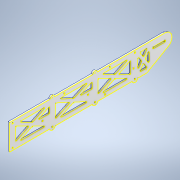
# Autodesk Inventor part: plyta_glowna_odchudzona
Saved by Autodesk Inventor 2022 (Build 260153000, 153)
## iProperties
Created: 2021-04-10
Part Number: plyta_glowna_odchudzona
Material: Aluminium 6061
Document SubType Name: Modeling
Designer: patryk.szydlik
Density: 2.7 g/cm^3
Appearance: Aluminium — płaski
Mass: 531.743 g
Surface Area: 1004.37 cm^2
Volume: 196.942 cm^3
Author: patryk.szydlik
Autodesk Inventor part; units mm, degrees
(part 1 of 2)
ref_plane "YZ Plane" through (0, 0, 0) normal (1, 0, 0) x (0, 1, 0)
ref_plane "XZ Plane" through (0, 0, 0) normal (0, 1, 0) x (-1, 0, 0)
ref_plane "XY Plane" through (0, 0, 0) normal (0, 0, 1) x (1, 0, 0)
sketch "Sketch2" plane through (0, 0, 0) normal (1, 0, 0) x (0, 1, 0)
  line L0 (127.2876, 96.9132) -> (-12.7124, 96.9132) construction
  line L1 (-12.7124, 96.9132) -> (-12.7124, -363.0868) construction
  line L2 (-12.7124, -363.0868) -> (127.2876, -363.0868) construction
  line L3 (127.2876, -363.0868) -> (127.2876, 96.9132) construction
  line L4 (97.2876, 66.9132) -> (17.2876, 66.9132) construction
  line L5 (17.2876, 66.9132) -> (17.2876, -333.0868) construction
  line L6 (17.2876, -333.0868) -> (97.2876, -333.0868) construction
  line L7 (97.2876, -333.0868) -> (97.2876, 66.9132) construction
  point P0 (0, 0)
  dimension "d2" = 140
  dimension "d3" = 460
  dimension "d4" = 80
  dimension "d5" = 400
  dimension "d6" = 30
  dimension "d7" = 30
  constraints: 16 end point, 4 parallel, 2 horizontal, 2 perpendicular
  measures "d2" distance of L2.end L1.end
  measures "d3" distance of L1.end L0.end
  measures "d4" distance of L6.end L5.end
  measures "d5" distance of L5.end L4.end
  measures "d6" distance between parallel lines of L3 L7
  measures "d7" distance between parallel lines of L0 L4
sketch "Sketch3" plane through (0, 0, 0) normal (1, 0, 0) x (0, 1, 0)
  circle A0 centre (-62.7124, 46.9132) radius 20
  line L0 (-12.7124, 96.9132) -> (-12.7124, -363.0868) construction
  circle A1 centre (-62.7124, -33.0868) radius 20
  circle A2 centre (-62.7124, -113.0868) radius 20
  circle A3 centre (-62.7124, -193.0868) radius 20
  circle A4 centre (-62.7124, -273.0868) radius 20
  circle A5 centre (-62.7124, -353.0868) radius 20
  line L1 (127.2876, 96.9132) -> (-12.7124, 96.9132) construction
  point P0 (0, 0)
  dimension "d8" = 40
  dimension "d9" = 50
  dimension "d12" = 80
  dimension "d17" = 50
  constraints: 6 centre point, 1 vertical, 10 other
  measures "d8" diameter of A0
  measures "d9" distance from line of L0 A0.centre
  measures "d12" distance of A0.centre A1.centre
  measures "d17" distance from line of A0.centre L1
sketch "Sketch1" plane through (0, 0, 0) normal (1, 0, 0) x (0, 1, 0)
  circle A0 centre (65.5719, 146.9132) radius 40
  circle A1 centre (65.5719, -453.0868) radius 40
  line L0 (127.2876, 96.9132) -> (-12.7124, 96.9132) construction
  line L1 (-12.7124, -363.0868) -> (127.2876, -363.0868) construction
  line L2 (-62.7124, 46.9132) -> (-62.7124, -33.0868) construction
  line L3 (-62.7124, -273.0868) -> (-62.7124, -353.0868) construction
  line L4 (105.2399, 141.7706) -> (105.5719, -453.0645) construction
  circle A2 centre (-62.7124, 46.9132) radius 20 projected
  line L5 (37.2876, 175.1975) -> (-76.8545, 61.0553)
  circle A3 centre (-62.7124, -353.0868) radius 20 projected
  line L6 (-76.8545, -367.2289) -> (37.2876, -481.3711) construction
  point P0 (0, 0)
  dimension "d0" = 80
  dimension "d1" = 80
  dimension "d18" = 50
  dimension "d19" = 90
  dimension "d45" = 135
  dimension "d46" = 135
  constraints: 10 end point, 4 point on circle, 3 tangent, 2 centre point, 2 coincident, 2 vertical, 6 other
  measures "d0" diameter of A0
  measures "d1" diameter of A1
  measures "d18" distance from line of A0.centre L0
  measures "d19" distance from line of A1.centre L1
  measures "d45" angle of L2 L5
  measures "d46" angle of L3 L6
sketch "Sketch4" plane through (0, 0, 0) normal (1, 0, 0) x (0, 1, 0)
  line L0 (37.6815, -23.0868) -> (-57.7124, 6.9132) construction
  circle A0 centre (-62.7124, 46.9132) radius 20 projected
  circle A1 centre (-62.7124, -33.0868) radius 20 projected
  line L1 (-62.7124, 46.9132) -> (-62.7124, -33.0868) construction
  circle A2 centre (-27.7124, 92.5679) radius 20 construction
  circle A3 centre (-27.7124, 12.5679) radius 20 construction
  line L2 (-27.7124, 52.5679) -> (37.6815, -23.0868) construction
  line L3 (-27.7124, 52.5679) -> (-57.7124, 6.9132) construction
  line L4 (37.6815, -23.0868) -> (-42.7124, 29.7406) construction
  line L5 (-12.7124, 96.9132) -> (-12.7124, -363.0868) construction
  point P0 (0, 0)
  point P1 (-61.7124, 47.9132)
  point P2 (83.0715, 59.9132)
  point P3 (83.0715, -100.0868)
  point P4 (37.6815, -183.0868)
  point P5 (83.0715, -260.0868)
  point P6 (37.6815, -343.0868)
  dimension "d22" = 40
  dimension "d23" = 5
  dimension "d24" = 30
  dimension "d25" = 40
  dimension "d26" = 40
  dimension "d27" = 80
  dimension "d28" = 40
  dimension "d29" = 100
  dimension "d30" = 100
  dimension "d31" = 35
  dimension "d32" = 54.6292
  dimension "d33" = 27.3146
  dimension "d34" = 56.691
  dimension "d35" = 95.3939
  dimension "d36" = 45.39
  dimension "d37" = 83
  dimension "d40" = 160
  constraints: 8 end point, 2 centre point, 2 vertical alignment, 1 coincident, 1 midpoint, 1 vertical, 4 other
  measures "d22" vertical distance of point (-62.712, 46.913) L0.end
  measures "d23" horizontal distance of point (-62.712, 46.913) L0.end
  measures "d24" vertical distance of L0.end L0.start
  measures "d25" diameter of A3
  measures "d26" diameter of A2
  measures "d27" distance of A3.centre A2.centre
  measures "d28" distance of A3.centre L2.start
  measures "d29" distance of L0.start L0.end
  measures "d30" distance of L2.start L0.start
  measures "d31" horizontal distance of point (-62.712, 46.913) A2.centre
  measures "d32" distance of L0.end L2.start
  measures "d33" distance of L0.end L4.end
  measures "d34" angle of L5 L4
  measures "d35" horizontal distance of L0.end L0.start
  measures "d36" horizontal distance of L0.start point (83.072, 59.913)
  measures "d37" vertical distance of L0.start point (83.072, 59.913)
  measures "d40" distance of point (83.072, 59.913) point (83.072, -100.087)
sketch "Sketch6" plane through (0, 0, 0) normal (1, 0, 0) x (0, 1, 0)
  line L0 (234.6261, -208.0868) -> (-157.479, -208.0868) construction
  line L1 (237.7494, -58.0868) -> (-154.3557, -58.0868) construction
  line L2 (17.2876, -333.0868) -> (97.2876, -333.0868) construction
  line L3 (97.2876, 66.9132) -> (17.2876, 66.9132) construction
  point P0 (0, 0)
  dimension "d61" = 125
  dimension "d62" = 125
  constraints: 4 end point, 2 horizontal
  measures "d61" distance between parallel lines of L1 L3
  measures "d62" distance between parallel lines of L2 L0
sketch "Sketch5" plane through (0, 0, 0) normal (1, 0, 0) x (0, 1, 0)
  arc A0 (90.5719, 146.9132) -> (47.8942, 164.5909) centre (65.5719, 146.9132) ccw
  arc A1 (90.5719, -453.0868) -> (43.9213, -465.5868) centre (65.5719, -453.0868) ccw construction
  line L0 (90.5719, -453.0868) -> (90.5719, 146.9132)
  arc A2 (30.1815, -170.0964) -> (23.5862, -188.2171) centre (37.6815, -183.0868) ccw
  arc A3 (30.1815, -330.0964) -> (23.5862, -348.2171) centre (37.6815, -343.0868) ccw
  arc A4 (30.1815, -10.0964) -> (22.6815, -23.0868) centre (37.6815, -23.0868) ccw
  line L1 (30.1815, -170.0964) -> (40.5719, -164.0975) construction
  line L2 (30.1815, -10.0964) -> (40.5719, -4.0975) construction
  circle A5 centre (83.0715, -100.0868) radius 12.5 construction
  circle A6 centre (83.0715, -260.0868) radius 12.5 construction
  circle A7 centre (83.0715, 59.9132) radius 12.5 construction
  line L3 (71.9467, 54.2134) -> (71.9467, 54.182) construction
  line L4 (72.2462, 53.6632) -> (71.9467, 54.182) construction
  line L5 (37.6815, -23.0868) -> (69.2216, -23.0868) construction
  arc A8 (47.8942, 164.5909) -> (90.5719, 146.9132) centre (65.5719, 146.9132) ccw construction
  arc A9 (40.5719, -8.3679) -> (30.1815, -10.0964) centre (37.6815, -23.0868) ccw construction
  arc A10 (40.5719, -37.8057) -> (40.5719, -8.3679) centre (37.6815, -23.0868) ccw construction
  arc A11 (22.6815, -23.0868) -> (40.5719, -37.8057) centre (37.6815, -23.0868) ccw construction
  arc A12 (40.5719, -168.3679) -> (30.1815, -170.0964) centre (37.6815, -183.0868) ccw construction
  arc A13 (40.5719, -197.8057) -> (40.5719, -168.3679) centre (37.6815, -183.0868) ccw construction
  arc A14 (23.5862, -188.2171) -> (40.5719, -197.8057) centre (37.6815, -183.0868) ccw construction
  arc A15 (40.5719, -328.3679) -> (30.1815, -330.0964) centre (37.6815, -343.0868) ccw construction
  arc A16 (23.5862, -348.2171) -> (40.5719, -328.3679) centre (37.6815, -343.0868) ccw construction
  arc A17 (43.9213, -465.5868) -> (90.5719, -453.0868) centre (65.5719, -453.0868) ccw
  arc A18 (62.5719, -453.0868) -> (68.5719, -453.0868) centre (65.5719, -453.0868) ccw
  arc A19 (68.5719, -413.0868) -> (62.5719, -413.0868) centre (65.5719, -413.0868) ccw
  line L6 (68.5719, -413.0868) -> (68.5719, -453.0868)
  line L7 (62.5719, -413.0868) -> (62.5719, -453.0868)
  arc A20 (68.5719, -453.0868) -> (62.5719, -453.0868) centre (65.5719, -453.0868) ccw construction
  arc A21 (62.5719, -413.0868) -> (68.5719, -413.0868) centre (65.5719, -413.0868) ccw construction
  line L8 (127.2876, 96.9132) -> (-12.7124, 96.9132) construction
  line L9 (-12.7124, -363.0868) -> (127.2876, -363.0868) construction
  line L10 (237.7494, -58.0868) -> (-154.3557, -58.0868) construction
  line L11 (234.6261, -208.0868) -> (-157.479, -208.0868) construction
  circle A22 centre (65.5719, 146.9132) radius 11
  circle A23 centre (65.5719, -413.0868) radius 50 construction
  circle A24 centre (65.5719, 146.9132) radius 55 construction
  line L12 (0.5719, 117.2685) -> (47.8942, 164.5909)
  line L13 (43.9213, -465.5868) -> (0.5719, -390.5035)
  line L14 (0.5719, -390.5035) -> (0.5719, 117.2685)
  line L15 (17.2876, 66.9132) -> (17.2876, -333.0868) construction
  circle A25 centre (2.2876, -58.0868) radius 10
  circle A26 centre (2.2876, -348.0868) radius 10
  circle A27 centre (2.2876, -208.0868) radius 10
  circle A28 centre (90.5719, -208.0868) radius 7.5
  circle A29 centre (90.5719, -58.0868) radius 7.5
  point P0 (0, 0)
  point P1 (71.9467, -17.6422)
  point P2 (71.9467, -177.6422)
  point P3 (71.9467, -268.3281)
  point P4 (71.9467, -337.6422)
  point P5 (83.0719, 81.9132)
  point P6 (83.0719, -348.0868)
  point P7 (83.0719, -366.2493)
  point P8 (16.3278, 122.4179)
  point P9 (16.56, -403.1957)
  point P10 (8.0719, -82.4742)
  point P11 (8.0719, -243.0868)
  point P12 (0.5719, -338.2351)
  point P13 (0.5719, -357.9385)
  point P14 (0.5719, -48.2351)
  point P15 (0.5719, -67.9385)
  point P16 (0.5719, -198.2351)
  point P17 (0.5719, -217.9385)
  point P18 (8.0719, 81.9132)
  point P19 (90.5719, -200.5868)
  point P20 (90.5719, -215.5868)
  point P21 (90.5719, -50.5868)
  point P22 (90.5719, -65.5868)
  dimension "d84" = 110
  dimension "d47" = 50
  dimension "d48" = 50
  dimension "d49" = 30
  dimension "d50" = 30
  dimension "d51" = 30
  dimension "d52" = 25
  dimension "d54" = 25
  dimension "d58" = 6
  dimension "d59" = 6
  dimension "d60" = 40
  dimension "d63" = 15
  dimension "d64" = 7.5
  dimension "d65" = 15
  dimension "d66" = 7.5
  dimension "d81" = 22
  dimension "d82" = 100
  dimension "d86" = 90
  dimension "d92" = 7.5
  dimension "d101" = 7.5
  dimension "d102" = 7.5
  dimension "d103" = 135
  dimension "d104" = 150
  dimension "d139" = 7.5004
  dimension "d141" = 0
  dimension "d142" = 0
  dimension "d145" = 25
  dimension "d150" = 15
  dimension "d151" = 15
  dimension "d152" = 20
  dimension "d153" = 20
  dimension "d154" = 20
  dimension "d155" = 15
  dimension "d159" = 15
  dimension "d160" = 7.5
  dimension "d161" = 15
  dimension "d162" = 15
  constraints: 45 point on circle, 29 centre point, 22 end point, 18 coincident, 8 point on line, 8 tangent, 4 vertical, 2 vertical alignment, 1 horizontal, 1 horizontal alignment, 3 other
  measures "d47" diameter of A0
  measures "d48" diameter of A1
  measures "d49" diameter of A2
  measures "d50" diameter of A3
  measures "d51" diameter of A4
  measures "d52" diameter of A5
  measures "d54" diameter of A7
  measures "d58" diameter of A18
  measures "d59" diameter of A19
  measures "d60" distance of point (65.572, -453.087) point (65.572, -413.087)
  measures "d63" distance from line of L8 point (83.072, 81.913)
  measures "d64" distance from line of L0 point (83.072, 81.913)
  measures "d65" distance from line of L9 point (83.072, -348.087)
  measures "d66" distance from line of L0 point (83.072, -348.087)
  measures "d81" diameter of A22
  measures "d82" diameter of A23
  measures "d86" distance between parallel lines of L14 L0
  measures "d92" distance from line of L0 A23.start
  measures "d101" distance from line of point (16.328, 122.418) L12
  measures "d102" distance from line of L13 A23.end
  measures "d103" angle of L12 L14
  measures "d104" angle of L14 L13
  measures "d139" distance from line of L0 point (83.072, -100.087)
  measures "d141" distance from line of L0 point (90.572, -58.087)
  measures "d142" distance from line of L0 point (90.572, -208.087)
  measures "d145" diameter of A6
  measures "d150" distance from line of point (2.288, -348.087) L15
  measures "d151" distance from line of L15 point (2.288, -58.087)
  measures "d152" diameter of A25
  measures "d153" diameter of A26
  measures "d154" diameter of A27
  measures "d155" distance from line of L15 point (2.288, -208.087)
  measures "d159" distance from line of L8 point (8.072, 81.913)
  measures "d160" distance from line of L14 point (8.072, 81.913)
  measures "d161" diameter of A28
  measures "d162" diameter of A29
extrude "Extrusion1" add sketch "Sketch5" against normal blind 5
hole "Hole1" at (0, 83.0719, 81.9132) at (0, 83.0715, 59.9132) at (0, 16.3278, 122.4179) at (0, 37.6815, -23.0868) at (0, 90.5719, -58.0868) at (0, 8.0719, -82.4742) at (0, 83.0715, -100.0868) at (0, 37.6815, -183.0868) at (0, 90.5719, -208.0868) at (0, 8.0719, -243.0868) at (0, 83.0715, -260.0868) at (0, 2.2876, -348.0868) at (0, 37.6815, -343.0868) at (0, 16.56, -403.1957) at (0, 83.0719, -348.0868) at (0, 83.0719, -366.2493) at (0, 2.2876, -58.0868) at (0, 2.2876, -208.0868) at (0, 8.0719, 81.9132) direction (-1, 0, 0) diameter 5 end through all clearance for "Flat Head Machine Screw" size "M5" standard "Ansi Metric M Profile"
sketch "Sketch7" plane through (0, 0, 0) normal (1, 0, 0) x (0, 0, -1)
  circle A0 centre (348.0868, 83.0719) radius 2.5 projected
  circle A1 centre (343.0868, 37.6815) radius 2.5 projected
  circle A2 centre (243.0868, 8.0719) radius 2.5 projected
  circle A3 centre (82.4742, 8.0719) radius 2.5 projected
  circle A4 centre (58.0868, 90.5719) radius 2.5 projected
  circle A5 centre (-122.4179, 16.3278) radius 2.5 projected
  circle A6 centre (-81.9132, 83.0719) radius 2.5 projected
  circle A7 centre (-59.9132, 83.0715) radius 2.5 projected
  circle A8 centre (23.0868, 37.6815) radius 2.5 projected
  circle A9 centre (100.0868, 83.0715) radius 2.5 projected
  circle A10 centre (183.0868, 37.6815) radius 2.5 projected
  circle A11 centre (208.0868, 90.5719) radius 2.5 projected
  circle A12 centre (260.0868, 83.0715) radius 2.5 projected
  circle A13 centre (348.0868, 2.2876) radius 2.5 projected
  circle A14 centre (403.1957, 16.56) radius 2.5 projected
  circle A15 centre (366.2493, 83.0719) radius 2.5 projected
  line L0 (-117.2685, 0.5719) -> (48.2351, 0.5719) projected
  line L1 (390.5035, 0.5719) -> (465.5868, 43.9213) projected
  arc A16 (465.5868, 43.9213) -> (453.0868, 90.5719) centre (453.0868, 65.5719) ccw projected
  line L2 (453.0868, 90.5719) -> (215.5868, 90.5719) projected
  arc A17 (-146.9132, 90.5719) -> (-164.5909, 47.8942) centre (-146.9132, 65.5719) ccw projected
  line L3 (-164.5909, 47.8942) -> (-117.2685, 0.5719) projected
  circle A18 centre (-146.9132, 65.5719) radius 11 projected
  arc A19 (453.0868, 62.5719) -> (453.0868, 68.5719) centre (453.0868, 65.5719) ccw projected
  line L4 (453.0868, 62.5719) -> (413.0868, 62.5719) projected
  arc A20 (413.0868, 68.5719) -> (413.0868, 62.5719) centre (413.0868, 65.5719) ccw projected
  line L5 (413.0868, 68.5719) -> (453.0868, 68.5719) projected
  line L6 (-146.9132, 75.5719) -> (453.0868, 75.5719)
  arc A21 (458.0868, 56.9116) -> (453.0868, 75.5719) centre (453.0868, 65.5719) ccw
  line L7 (458.0868, 56.9116) -> (386.4843, 15.5719)
  line L8 (386.4843, 15.5719) -> (398.0868, 15.5719)
  line L9 (-111.0553, 15.5719) -> (-153.9843, 58.5008)
  arc A22 (-146.9132, 75.5719) -> (-153.9843, 58.5008) centre (-146.9132, 65.5719) ccw
  line L10 (453.0868, 90.5719) -> (-146.9132, 90.5719) projected
  line L11 (-91.9132, 90.5719) -> (-71.9132, 90.5719)
  line L12 (-71.9132, 90.5719) -> (-71.9132, 0.5719)
  line L13 (-71.9132, 0.5719) -> (-91.9132, 0.5719)
  line L14 (-91.9132, 0.5719) -> (-91.9132, 90.5719)
  line L15 (-117.2685, 0.5719) -> (390.5035, 0.5719) projected
  line L16 (48.0868, 90.5719) -> (68.0868, 90.5719)
  line L17 (68.0868, 90.5719) -> (68.0868, 0.5719)
  line L18 (68.0868, 0.5719) -> (48.0868, 0.5719)
  line L19 (48.0868, 0.5719) -> (48.0868, 90.5719)
  line L20 (198.0868, 90.5719) -> (218.0868, 90.5719)
  line L21 (218.0868, 90.5719) -> (218.0868, 0.5719)
  line L22 (218.0868, 0.5719) -> (198.0868, 0.5719)
  line L23 (198.0868, 0.5719) -> (198.0868, 90.5719)
  line L24 (338.0868, 90.5719) -> (358.0868, 90.5719)
  line L25 (358.0868, 90.5719) -> (358.0868, 38.7436)
  line L26 (358.0868, 0.5719) -> (338.0868, 0.5719)
  line L27 (338.0868, 0.5719) -> (338.0868, 90.5719)
  circle A23 centre (-146.9132, 65.5719) radius 25 construction
  arc A24 (453.0868, 62.5719) -> (453.0868, 68.5719) centre (453.0868, 65.5719) ccw construction
  circle A25 centre (453.0868, 65.5719) radius 25 construction
  arc A26 (413.0868, 68.5719) -> (413.0868, 62.5719) centre (413.0868, 65.5719) ccw construction
  line L28 (-146.9132, 90.5719) -> (453.0868, 90.5719) construction
  line L29 (398.0911, 65.9314) -> (398.0911, 90.5719) construction
  line L30 (403.0868, 38.7436) -> (456.6188, 38.7436) construction
  line L31 (465.5868, 43.9213) -> (390.5035, 0.5719) construction
  line L32 (403.0868, 38.7436) -> (403.0868, 15.5719) construction
  line L33 (398.0868, 65.5719) -> (398.0868, 38.7436) construction
  line L34 (398.0868, 38.7436) -> (398.0868, 38.7436) construction
  line L35 (398.0868, 15.5719) -> (398.0868, 38.7436) construction
  line L36 (408.0868, 38.7436) -> (408.0868, 15.5719) construction
  line L37 (358.0868, 38.7436) -> (358.0868, 0.5719)
  line L38 (398.0868, 38.7436) -> (403.0868, 38.7436) construction
  line L39 (398.0868, 15.5719) -> (-111.0553, 15.5719)
  line L40 (218.0868, 75.5719) -> (338.0868, 15.5719) construction
  line L41 (218.0868, 15.5719) -> (338.0868, 75.5719) construction
  line L42 (326.9065, 75.5719) -> (218.0868, 21.1621) construction
  line L43 (229.2671, 15.5719) -> (338.0868, 69.9817) construction
  line L44 (229.2671, 75.5719) -> (338.0868, 21.1621) construction
  line L45 (218.0868, 69.9817) -> (326.9065, 15.5719) construction
  line L46 (333.0868, 67.4817) -> (333.0868, 23.6621) construction
  line L47 (68.0868, 75.5719) -> (198.0868, 15.5719) construction
  line L48 (198.0868, 75.5719) -> (68.0868, 15.5719) construction
  line L49 (68.0868, 21.0788) -> (186.1553, 75.5719) construction
  line L50 (80.0183, 15.5719) -> (198.0868, 70.065) construction
  line L51 (198.0868, 21.0788) -> (80.0183, 75.5719) construction
  line L52 (68.0868, 70.065) -> (186.1553, 15.5719) construction
  line L53 (48.0868, 15.5719) -> (-71.9132, 75.5719) construction
  line L54 (-71.9132, 15.5719) -> (48.0868, 75.5719) construction
  line L55 (36.9065, 75.5719) -> (-71.9132, 21.1621) construction
  line L56 (-60.7329, 15.5719) -> (48.0868, 69.9817) construction
  line L57 (-60.7329, 75.5719) -> (48.0868, 21.1621) construction
  line L58 (-71.9132, 69.9817) -> (36.9065, 15.5719) construction
  line L59 (68.0868, 73.0715) -> (61.5727, 73.0715) construction
  line L60 (48.0868, 47.6815) -> (-4.9522, 47.6815) construction
  line L61 (198.0868, 47.6815) -> (140.4474, 47.6815) construction
  line L62 (218.0868, 73.0715) -> (211.9072, 73.0715) construction
  line L63 (-121.9132, 65.5719) -> (-121.9132, 75.5719) construction
  line L64 (-121.9132, 65.5719) -> (-121.9132, 26.4298) construction
  line L65 (-121.9132, 75.5719) -> (-91.9132, 15.5719) construction
  line L66 (-91.9132, 26.7522) -> (-116.323, 75.5719) construction
  line L67 (-121.9132, 64.3916) -> (-97.5034, 15.5719) construction
  line L68 (-111.0553, 15.5719) -> (-121.9132, 15.5719) construction
  line L69 (-121.9132, 15.5719) -> (-121.9132, 26.4298) construction
  line L70 (-121.9132, 15.5719) -> (-91.9132, 75.5719) construction
  line L71 (-97.5034, 75.5719) -> (-121.9132, 26.7522) construction
  line L72 (-116.323, 15.5719) -> (-91.9132, 64.3916) construction
  circle A27 centre (413.0868, 65.5719) radius 15 construction
  line L73 (398.0911, 75.5719) -> (358.0868, 15.5719) construction
  line L74 (398.0868, 15.5719) -> (358.0868, 75.5719) construction
  line L75 (392.0816, 75.5719) -> (358.0868, 24.5851) construction
  line L76 (398.0911, 66.5587) -> (364.0962, 15.5719) construction
  line L77 (358.0868, 66.558) -> (392.0775, 15.5719) construction
  line L78 (398.0868, 24.5858) -> (364.096, 75.5719) construction
  circle A28 centre (58.0868, 2.2876) radius 2.5 projected
  line L79 (67.9385, 0.5719) -> (198.2351, 0.5719) projected
  line L80 (217.9385, 0.5719) -> (338.2351, 0.5719) projected
  arc A29 (48.2351, 0.5719) -> (67.9385, 0.5719) centre (58.0868, 2.2876) ccw projected
  arc A30 (338.2351, 0.5719) -> (357.9385, 0.5719) centre (348.0868, 2.2876) ccw projected
  arc A31 (198.2351, 0.5719) -> (217.9385, 0.5719) centre (208.0868, 2.2876) ccw projected
  line L81 (357.9385, 0.5719) -> (390.5035, 0.5719) projected
  line L82 (200.5868, 90.5719) -> (65.5868, 90.5719) projected
  line L83 (50.5868, 90.5719) -> (-146.9132, 90.5719) projected
  arc A32 (215.5868, 90.5719) -> (200.5868, 90.5719) centre (208.0868, 90.5719) ccw projected
  arc A33 (65.5868, 90.5719) -> (50.5868, 90.5719) centre (58.0868, 90.5719) ccw projected
  point P0 (0, 0)
  dimension "d93" = 15
  dimension "d94" = 10
  dimension "d95" = 20
  dimension "d97" = 20
  dimension "d99" = 20
  dimension "d100" = 10
  dimension "d105" = 20
  dimension "d107" = 5
  dimension "d108" = 5
  dimension "d111" = 5
  dimension "d112" = 5
  dimension "d113" = 5
  dimension "d114" = 5
  dimension "d115" = 10
  dimension "d116" = 5
  dimension "d117" = 5
  dimension "d118" = 5
  dimension "d119" = 5
  dimension "d120" = 5
  dimension "d121" = 5
  dimension "d122" = 5
  dimension "d123" = 5
  dimension "d124" = 10
  dimension "d125" = 10
  dimension "d126" = 10
  dimension "d127" = 10
  dimension "d128" = 5
  dimension "d129" = 5
  dimension "d130" = 5
  dimension "d131" = 5
  dimension "d132" = 30
  dimension "d133" = 5
  dimension "d134" = 5
  dimension "d135" = 5
  dimension "d136" = 5
  dimension "d148" = 10
  dimension "d149" = 10
  constraints: 134 end point, 61 point on line, 29 parallel, 11 perpendicular, 9 horizontal, 6 point on circle, 6 vertical, 4 centre point, 4 coincident, 1 collinear, 1 concentric, 1 horizontal alignment, 50 other
  measures "d94" distance from line of L12 A6.centre
  measures "d95" distance of L17.end L18.end
  measures "d97" distance of L21.end L22.end
  measures "d99" distance of L26.start L26.end
  measures "d100" distance from line of L25 A0.centre
  measures "d105" distance between parallel lines of L12 L14
  measures "d107" distance between parallel lines of L35 L32
  measures "d108" distance between parallel lines of L32 L36
  measures "d111" distance between parallel lines of L42 L41
  measures "d112" distance between parallel lines of L41 L43
  measures "d113" distance between parallel lines of L40 L44
  measures "d114" distance between parallel lines of L45 L40
  measures "d115" distance from line of L46 A1.centre
  measures "d116" distance between parallel lines of L50 L48
  measures "d117" distance between parallel lines of L49 L48
  measures "d118" distance between parallel lines of L51 L47
  measures "d119" distance between parallel lines of L52 L47
  measures "d120" distance between parallel lines of L57 L53
  measures "d121" distance between parallel lines of L58 L53
  measures "d122" distance between parallel lines of L54 L55
  measures "d123" distance between parallel lines of L56 L54
  measures "d124" distance from line of L59 A9.centre
  measures "d125" distance from line of L60 A8.centre
  measures "d126" distance from line of L61 A10.centre
  measures "d127" distance from line of L62 A12.centre
  measures "d128" distance between parallel lines of L65 L66
  measures "d129" distance between parallel lines of L65 L67
  measures "d130" distance between parallel lines of L72 L70
  measures "d131" distance between parallel lines of L71 L70
  measures "d132" diameter of A27
  measures "d133" distance between parallel lines of L73 L75
  measures "d134" distance between parallel lines of L76 L73
  measures "d135" distance between parallel lines of L78 L74
  measures "d136" distance between parallel lines of L77 L74
  measures "d148" distance from line of L17 A4.centre
  measures "d149" distance from line of L23 A11.centre
sketch "Sketch8" plane through (0, 0, 0) normal (1, 0, 0) x (0, 0, -1)
  line L0 (-116.323, 15.5719) -> (-91.9132, 64.3916) projected
  line L1 (-91.9132, 26.7522) -> (-116.323, 75.5719) projected
  line L2 (-91.9132, 0.5719) -> (-91.9132, 90.5719) projected
  line L3 (-121.9132, 64.3916) -> (-97.5034, 15.5719) projected
  line L4 (398.0868, 15.5719) -> (-111.0553, 15.5719) projected
  line L5 (-111.0553, 15.5719) -> (-121.9132, 15.5719) projected
  line L6 (-97.5034, 75.5719) -> (-121.9132, 26.7522) projected
  line L7 (-121.9132, 65.5719) -> (-121.9132, 26.4298) projected
  line L8 (-146.9132, 75.5719) -> (453.0868, 75.5719) projected
  line L9 (-71.9132, 69.9817) -> (36.9065, 15.5719) projected
  line L10 (-71.9132, 90.5719) -> (-71.9132, 0.5719) projected
  line L11 (36.9065, 75.5719) -> (-71.9132, 21.1621) projected
  line L12 (-60.7329, 75.5719) -> (48.0868, 21.1621) projected
  line L13 (-60.7329, 15.5719) -> (48.0868, 69.9817) projected
  line L14 (48.0868, 47.6815) -> (-4.9522, 47.6815) projected
  line L15 (48.0868, 0.5719) -> (48.0868, 90.5719) projected
  line L16 (68.0868, 73.0715) -> (61.5727, 73.0715) projected
  line L17 (68.0868, 90.5719) -> (68.0868, 0.5719) projected
  line L18 (68.0868, 21.0788) -> (186.1553, 75.5719) projected
  line L19 (80.0183, 15.5719) -> (198.0868, 70.065) projected
  line L20 (68.0868, 70.065) -> (186.1553, 15.5719) projected
  line L21 (198.0868, 21.0788) -> (80.0183, 75.5719) projected
  line L22 (198.0868, 47.6815) -> (140.4474, 47.6815) projected
  line L23 (198.0868, 0.5719) -> (198.0868, 90.5719) projected
  line L24 (218.0868, 73.0715) -> (211.9072, 73.0715) projected
  line L25 (218.0868, 69.9817) -> (326.9065, 15.5719) projected
  line L26 (326.9065, 75.5719) -> (218.0868, 21.1621) projected
  line L27 (218.0868, 90.5719) -> (218.0868, 0.5719) projected
  line L28 (229.2671, 15.5719) -> (338.0868, 69.9817) projected
  line L29 (229.2671, 75.5719) -> (338.0868, 21.1621) projected
  line L30 (333.0868, 67.4817) -> (333.0868, 23.6621) projected
  line L31 (358.0868, 66.558) -> (392.0775, 15.5719) projected
  line L32 (392.0816, 75.5719) -> (358.0868, 24.5851) projected
  line L33 (358.0868, 90.5719) -> (358.0868, 38.7436) projected
  line L34 (358.0868, 38.7436) -> (358.0868, 0.5719) projected
  line L35 (398.0911, 66.5587) -> (364.0962, 15.5719) projected
  line L36 (398.0868, 24.5858) -> (364.096, 75.5719) projected
  line L37 (398.0868, 65.5719) -> (398.0868, 38.7436) projected
  line L38 (398.0868, 15.5719) -> (398.0868, 38.7436) projected
  line L39 (386.4843, 15.5719) -> (398.0868, 15.5719) projected
  line L40 (398.0911, 66.5587) -> (398.0868, 24.5858)
  point P0 (0, 0)
  point P1 (408.0868, 38.7436)
  point P2 (408.0868, 15.5719)
  point P3 (378.0876, 36.5567)
  point P4 (378.0881, 54.5838)
  point P5 (372.0785, 45.5704)
  point P6 (278.0868, 51.1621)
  point P7 (289.2671, 45.5719)
  point P8 (278.0868, 39.9817)
  point P9 (266.9065, 45.5719)
  point P10 (133.0868, 51.0788)
  point P11 (149.5892, 47.6815)
  point P12 (133.0868, 40.065)
  point P13 (121.1553, 45.5719)
  point P14 (3.4864, 47.6815)
  point P15 (-11.9132, 39.9817)
  point P16 (-11.9132, 51.1621)
  point P17 (-23.0935, 45.5719)
  point P18 (-101.323, 45.5719)
  point P19 (-106.9132, 34.3916)
  point P20 (-106.9132, 56.7522)
  point P21 (-112.5034, 45.5719)
  point P22 (384.0972, 45.5701)
  constraints: 2 end point, 2 other
extrude "Extrusion2" cut sketch "Sketch8" against normal blind 5 contours L6 L7 L3 | L0 L3 L4 L5 | L0 L2 L1 | L1 L8 L6 | L13 L9 L4 | L10 L9 L11 | L8 L11 L12 | L13 L15 L14 | L19 L20 L4 | L17 L20 L18 | L8 L18 L21 | L19 L23 L22 | L28 L25 L4 | L27 L25 L26 | L8 L26 L29 | L28 L30 L29 | L35 L31 L4 | L34 L33 L31 L32 | L8 L32 L36 | L35 L40 L38 L36
fillet "Zaokrąglenie1" radius 10 1 edges at (-2.5, 0.5719, 117.2685)
fillet "Zaokrąglenie2" radius 10 1 edges at (-2.5, 0.5719, -390.5035)
fillet "Zaokrąglenie3" radius 2 60 edges at (-2.5, 75.5719, 116.323) (-2.5, 15.5719, 116.323) (-2.5, 34.3916, 106.9132) (-2.5, 26.7522, 121.9132) (-2.5, 64.3916, 121.9132) (-2.5, 45.5719, 112.5034) (-2.5, 45.5719, 101.323) (-2.5, 15.5719, 97.5034) (-2.5, 64.3916, 91.9132) (-2.5, 56.7522, 106.9132) (-2.5, 75.5719, 97.5034) (-2.5, 26.7522, 91.9132) (-2.5, 69.9817, 71.9132) (-2.5, 75.5719, 60.7329) (-2.5, 45.5719, 23.0935) (-2.5, 47.6815, -3.4864) (-2.5, 51.1621, 11.9132) (-2.5, 39.9817, 11.9132) (-2.5, 15.5719, 60.7329) (-2.5, 21.1621, 71.9132) (-2.5, 69.9817, -48.0868) (-2.5, 47.6815, -48.0868) (-2.5, 15.5719, -36.9065) (-2.5, 75.5719, -36.9065) (-2.5, 70.065, -68.0868) (-2.5, 75.5719, -80.0183) (-2.5, 45.5719, -121.1553) (-2.5, 21.0788, -68.0868) (-2.5, 15.5719, -80.0183) (-2.5, 47.6815, -149.5892) (-2.5, 51.0788, -133.0868) (-2.5, 40.065, -133.0868) (-2.5, 75.5719, -186.1553) (-2.5, 70.065, -198.0868) (-2.5, 47.6815, -198.0868) (-2.5, 15.5719, -186.1553) (-2.5, 21.1621, -218.0868) (-2.5, 15.5719, -229.2671) (-2.5, 69.9817, -218.0868) (-2.5, 75.5719, -229.2671) (-2.5, 51.1621, -278.0868) (-2.5, 39.9817, -278.0868) (-2.5, 45.5719, -266.9065) (-2.5, 45.5719, -289.2671) (-2.5, 75.5719, -326.9065) (-2.5, 67.4817, -333.0868) (-2.5, 23.6621, -333.0868) (-2.5, 15.5719, -326.9065) (-2.5, 24.5851, -358.0868) (-2.5, 15.5719, -364.0962) (-2.5, 36.5567, -378.0876) (-2.5, 15.5719, -392.0775) (-2.5, 24.5858, -398.0868) (-2.5, 66.5587, -398.0911) (-2.5, 45.5701, -384.0972) (-2.5, 45.5704, -372.0785) (-2.5, 66.558, -358.0868) (-2.5, 75.5719, -364.096) (-2.5, 75.5719, -392.0816) (-2.5, 54.5838, -378.0881)
sketch "Sketch9" plane through (0, 0, 0) normal (1, 0, 0) x (0, 0, -1)
  line L0 (394.4234, 30.0809) -> (384.8369, 44.4607) projected
  arc A0 (384.8369, 46.6796) -> (384.8369, 44.4607) centre (386.501, 45.5701) ccw projected
  line L1 (384.8369, 46.6796) -> (394.4264, 61.0622) projected
  arc A1 (398.0904, 59.9525) -> (394.4264, 61.0622) centre (396.0904, 59.9527) ccw projected
  line L2 (398.0904, 59.9525) -> (398.0875, 31.1901) projected
  arc A2 (394.4234, 30.0809) -> (398.0875, 31.1901) centre (396.0875, 31.1903) ccw projected
  line L3 (-95.7021, 34.3299) -> (-100.8758, 44.6775) projected
  arc A3 (-100.8758, 46.4663) -> (-100.8758, 44.6775) centre (-99.087, 45.5719) ccw projected
  line L4 (-100.8758, 46.4663) -> (-95.7021, 56.8138) projected
  arc A4 (-91.9132, 55.9194) -> (-95.7021, 56.8138) centre (-93.9132, 55.9194) ccw projected
  line L5 (-91.9132, 55.9194) -> (-91.9132, 35.2244) projected
  arc A5 (-95.7021, 34.3299) -> (-91.9132, 35.2244) centre (-93.9132, 35.2244) ccw projected
  line L6 (46.0868, 47.6815) -> (11.9586, 47.6815) projected
  arc A6 (11.0641, 51.4704) -> (11.9586, 47.6815) centre (11.9586, 49.6815) ccw projected
  line L7 (11.0641, 51.4704) -> (45.1924, 68.5345) projected
  arc A7 (48.0868, 66.7457) -> (45.1924, 68.5345) centre (46.0868, 66.7457) ccw projected
  line L8 (48.0868, 66.7457) -> (48.0868, 49.6815) projected
  arc A8 (46.0868, 47.6815) -> (48.0868, 49.6815) centre (46.0868, 49.6815) ccw projected
  line L9 (278.9812, 39.5345) -> (319.3287, 19.3608) projected
  arc A9 (318.4343, 15.5719) -> (319.3287, 19.3608) centre (318.4343, 17.5719) ccw projected
  line L10 (318.4343, 15.5719) -> (237.7393, 15.5719) projected
  arc A10 (236.8448, 19.3608) -> (237.7393, 15.5719) centre (237.7393, 17.5719) ccw projected
  line L11 (236.8448, 19.3608) -> (277.1924, 39.5345) projected
  arc A11 (278.9812, 39.5345) -> (277.1924, 39.5345) centre (278.0868, 37.7457) ccw projected
  line L12 (367.8331, 75.5719) -> (388.3444, 75.5719) projected
  arc A12 (390.0084, 72.4624) -> (388.3444, 75.5719) centre (388.3444, 73.5719) ccw projected
  line L13 (390.0084, 72.4624) -> (379.7522, 57.0798) projected
  arc A13 (376.4241, 57.0798) -> (379.7522, 57.0798) centre (378.0882, 58.1892) ccw projected
  line L14 (376.4241, 57.0798) -> (366.169, 72.4625) projected
  arc A14 (367.8331, 75.5719) -> (366.169, 72.4625) centre (367.8331, 73.5719) ccw projected
  line L15 (361.7509, 61.0619) -> (371.3389, 46.6799) projected
  arc A15 (371.3388, 44.461) -> (371.3389, 46.6799) centre (369.6748, 45.5705) ccw projected
  line L16 (371.3388, 44.461) -> (361.7508, 30.0806) projected
  arc A16 (358.0868, 31.1901) -> (361.7508, 30.0806) centre (360.0868, 31.1901) ccw projected
  line L17 (358.0868, 31.1901) -> (358.0868, 59.9525) projected
  arc A17 (361.7509, 61.0619) -> (358.0868, 59.9525) centre (360.0868, 59.9525) ccw projected
  line L18 (89.1243, 75.5719) -> (177.0493, 75.5719) projected
  arc A18 (177.8875, 71.756) -> (177.0493, 75.5719) centre (177.0493, 73.5719) ccw projected
  line L19 (177.8875, 71.756) -> (133.9249, 51.4656) projected
  arc A19 (132.2487, 51.4656) -> (133.9249, 51.4656) centre (133.0868, 53.2815) ccw projected
  line L20 (132.2487, 51.4656) -> (88.2861, 71.756) projected
  arc A20 (89.1243, 75.5719) -> (88.2861, 71.756) centre (89.1243, 73.5719) ccw projected
  line L21 (-11.0188, 39.5345) -> (29.3287, 19.3608) projected
  arc A21 (28.4343, 15.5719) -> (29.3287, 19.3608) centre (28.4343, 17.5719) ccw projected
  line L22 (28.4343, 15.5719) -> (-52.2607, 15.5719) projected
  arc A22 (-53.1552, 19.3608) -> (-52.2607, 15.5719) centre (-52.2607, 17.5719) ccw projected
  line L23 (-53.1552, 19.3608) -> (-12.8076, 39.5345) projected
  arc A23 (-11.0188, 39.5345) -> (-12.8076, 39.5345) centre (-11.9132, 37.7457) ccw projected
  line L24 (-105.1244, 30.8138) -> (-98.9506, 18.4663) projected
  arc A24 (-100.7394, 15.5719) -> (-98.9506, 18.4663) centre (-100.7394, 17.5719) ccw projected
  line L25 (-100.7394, 15.5719) -> (-113.087, 15.5719) projected
  arc A25 (-114.8758, 18.4663) -> (-113.087, 15.5719) centre (-113.087, 17.5719) ccw projected
  line L26 (-114.8758, 18.4663) -> (-108.7021, 30.8138) projected
  arc A26 (-105.1244, 30.8138) -> (-108.7021, 30.8138) centre (-106.9132, 29.9194) ccw projected
  line L27 (117.2208, 43.756) -> (70.9249, 22.3887) projected
  arc A27 (68.0868, 24.2046) -> (70.9249, 22.3887) centre (70.0868, 24.2046) ccw projected
  line L28 (68.0868, 24.2046) -> (68.0868, 66.9392) projected
  arc A28 (70.9249, 68.7551) -> (68.0868, 66.9392) centre (70.0868, 66.9392) ccw projected
  line L29 (70.9249, 68.7551) -> (117.2208, 47.3878) projected
  arc A29 (117.2208, 43.756) -> (117.2208, 47.3878) centre (116.3827, 45.5719) ccw projected
  line L30 (-118.1244, 56.8138) -> (-112.9506, 46.4663) projected
  arc A30 (-112.9506, 44.6775) -> (-112.9506, 46.4663) centre (-114.7394, 45.5719) ccw projected
  line L31 (-112.9506, 44.6775) -> (-118.1244, 34.3299) projected
  arc A31 (-121.9132, 35.2244) -> (-118.1244, 34.3299) centre (-119.9132, 35.2244) ccw projected
  line L32 (-121.9132, 35.2244) -> (-121.9132, 55.9194) projected
  arc A32 (-118.1244, 56.8138) -> (-121.9132, 55.9194) centre (-119.9132, 55.9194) ccw projected
  line L33 (-71.9132, 24.3981) -> (-71.9132, 66.7457) projected
  arc A33 (-69.0188, 68.5345) -> (-71.9132, 66.7457) centre (-69.9132, 66.7457) ccw projected
  line L34 (-69.0188, 68.5345) -> (-26.6713, 47.3608) projected
  arc A34 (-26.6713, 43.783) -> (-26.6713, 47.3608) centre (-27.5657, 45.5719) ccw projected
  line L35 (-26.6713, 43.783) -> (-69.0188, 22.6093) projected
  arc A35 (-71.9132, 24.3981) -> (-69.0188, 22.6093) centre (-69.9132, 24.3981) ccw projected
  line L36 (177.0493, 15.5719) -> (89.1243, 15.5719) projected
  arc A36 (88.2861, 19.3878) -> (89.1243, 15.5719) centre (89.1243, 17.5719) ccw projected
  line L37 (88.2861, 19.3878) -> (132.2487, 39.6782) projected
  arc A37 (133.9249, 39.6782) -> (132.2487, 39.6782) centre (133.0868, 37.8623) ccw projected
  line L38 (133.9249, 39.6782) -> (177.8875, 19.3878) projected
  arc A38 (177.0493, 15.5719) -> (177.8875, 19.3878) centre (177.0493, 17.5719) ccw projected
  line L39 (330.1924, 25.1093) -> (292.8448, 43.783) projected
  arc A39 (292.8448, 47.3608) -> (292.8448, 43.783) centre (293.7393, 45.5719) ccw projected
  line L40 (292.8448, 47.3608) -> (330.1924, 66.0345) projected
  arc A40 (333.0868, 64.2457) -> (330.1924, 66.0345) centre (331.0868, 64.2457) ccw projected
  line L41 (333.0868, 64.2457) -> (333.0868, 26.8981) projected
  arc A41 (330.1924, 25.1093) -> (333.0868, 26.8981) centre (331.0868, 26.8981) ccw projected
  line L42 (379.7517, 34.0607) -> (390.0046, 18.6813) projected
  arc A42 (388.3405, 15.5719) -> (390.0046, 18.6813) centre (388.3405, 17.5719) ccw projected
  line L43 (388.3405, 15.5719) -> (367.8335, 15.5719) projected
  arc A43 (366.1695, 18.6814) -> (367.8335, 15.5719) centre (367.8335, 17.5719) ccw projected
  line L44 (366.1695, 18.6814) -> (376.4235, 34.0608) projected
  arc A44 (379.7517, 34.0607) -> (376.4235, 34.0608) centre (378.0876, 32.9513) ccw projected
  line L45 (237.7393, 75.5719) -> (318.4343, 75.5719) projected
  arc A45 (319.3287, 71.783) -> (318.4343, 75.5719) centre (318.4343, 73.5719) ccw projected
  line L46 (319.3287, 71.783) -> (278.9812, 51.6093) projected
  arc A46 (277.1924, 51.6093) -> (278.9812, 51.6093) centre (278.0868, 53.3981) ccw projected
  line L47 (277.1924, 51.6093) -> (236.8448, 71.783) projected
  arc A47 (237.7393, 75.5719) -> (236.8448, 71.783) centre (237.7393, 73.5719) ccw projected
  line L48 (196.0868, 47.6815) -> (158.6952, 47.6815) projected
  arc A48 (157.857, 51.4975) -> (158.6952, 47.6815) centre (158.6952, 49.6815) ccw projected
  line L49 (157.857, 51.4975) -> (195.2487, 68.7551) projected
  arc A49 (198.0868, 66.9392) -> (195.2487, 68.7551) centre (196.0868, 66.9392) ccw projected
  line L50 (198.0868, 66.9392) -> (198.0868, 49.6815) projected
  arc A50 (196.0868, 47.6815) -> (198.0868, 49.6815) centre (196.0868, 49.6815) ccw projected
  line L51 (-52.2607, 75.5719) -> (28.4343, 75.5719) projected
  arc A51 (29.3287, 71.783) -> (28.4343, 75.5719) centre (28.4343, 73.5719) ccw projected
  line L52 (29.3287, 71.783) -> (-11.0188, 51.6093) projected
  arc A52 (-12.8076, 51.6093) -> (-11.0188, 51.6093) centre (-11.9132, 53.3981) ccw projected
  line L53 (-12.8076, 51.6093) -> (-53.1552, 71.783) projected
  arc A53 (-52.2607, 75.5719) -> (-53.1552, 71.783) centre (-52.2607, 73.5719) ccw projected
  line L54 (-98.9506, 72.6775) -> (-105.1244, 60.3299) projected
  arc A54 (-108.7021, 60.3299) -> (-105.1244, 60.3299) centre (-106.9132, 61.2244) ccw projected
  line L55 (-108.7021, 60.3299) -> (-114.8758, 72.6775) projected
  arc A55 (-113.087, 75.5719) -> (-114.8758, 72.6775) centre (-113.087, 73.5719) ccw projected
  line L56 (-113.087, 75.5719) -> (-100.7394, 75.5719) projected
  arc A56 (-98.9506, 72.6775) -> (-100.7394, 75.5719) centre (-100.7394, 73.5719) ccw projected
  line L57 (220.9812, 68.5345) -> (263.3287, 47.3608) projected
  arc A57 (263.3287, 43.783) -> (263.3287, 47.3608) centre (262.4343, 45.5719) ccw projected
  line L58 (263.3287, 43.783) -> (220.9812, 22.6093) projected
  arc A58 (218.0868, 24.3981) -> (220.9812, 22.6093) centre (220.0868, 24.3981) ccw projected
  line L59 (218.0868, 24.3981) -> (218.0868, 66.7457) projected
  arc A59 (220.9812, 68.5345) -> (218.0868, 66.7457) centre (220.0868, 66.7457) ccw projected
  circle A60 centre (208.0868, 2.2876) radius 2.5 projected
  circle A61 centre (366.2493, 83.0719) radius 2.5 projected
  circle A62 centre (403.1957, 16.56) radius 2.5 projected
  circle A63 centre (348.0868, 2.2876) radius 2.5 projected
  circle A64 centre (243.0868, 8.0719) radius 2.5 projected
  circle A65 centre (183.0868, 37.6815) radius 2.5 projected
  circle A66 centre (82.4742, 8.0719) radius 2.5 projected
  circle A67 centre (23.0868, 37.6815) radius 2.5 projected
  circle A68 centre (-59.9132, 83.0715) radius 2.5 projected
  circle A69 centre (-81.9132, 83.0719) radius 2.5 projected
  circle A70 centre (-122.4179, 16.3278) radius 2.5 projected
  circle A71 centre (58.0868, 90.5719) radius 2.5 projected
  circle A72 centre (100.0868, 83.0715) radius 2.5 projected
  circle A73 centre (208.0868, 90.5719) radius 2.5 projected
  circle A74 centre (260.0868, 83.0715) radius 2.5 projected
  circle A75 centre (343.0868, 37.6815) radius 2.5 projected
  circle A76 centre (348.0868, 83.0719) radius 2.5 projected
  circle A77 centre (58.0868, 2.2876) radius 2.5 projected
  circle A78 centre (-81.9132, 8.0719) radius 2.5 projected
  arc A79 (387.824, 0.5719) -> (392.824, 1.9116) centre (387.824, 10.5719) ccw projected
  line L60 (392.824, 1.9116) -> (465.5868, 43.9213) projected
  arc A80 (465.5868, 43.9213) -> (453.0868, 90.5719) centre (453.0868, 65.5719) ccw projected
  line L61 (453.0868, 90.5719) -> (215.5868, 90.5719) projected
  arc A81 (215.5868, 90.5719) -> (200.5868, 90.5719) centre (208.0868, 90.5719) ccw projected
  line L62 (200.5868, 90.5719) -> (65.5868, 90.5719) projected
  arc A82 (65.5868, 90.5719) -> (50.5868, 90.5719) centre (58.0868, 90.5719) ccw projected
  line L63 (50.5868, 90.5719) -> (-146.9132, 90.5719) projected
  arc A83 (-146.9132, 90.5719) -> (-164.5909, 47.8942) centre (-146.9132, 65.5719) ccw projected
  line L64 (-164.5909, 47.8942) -> (-120.1975, 3.5008) projected
  arc A84 (-120.1975, 3.5008) -> (-113.1264, 0.5719) centre (-113.1264, 10.5719) ccw projected
  line L65 (-113.1264, 0.5719) -> (48.2351, 0.5719) projected
  arc A85 (48.2351, 0.5719) -> (67.9385, 0.5719) centre (58.0868, 2.2876) ccw projected
  line L66 (67.9385, 0.5719) -> (198.2351, 0.5719) projected
  arc A86 (198.2351, 0.5719) -> (217.9385, 0.5719) centre (208.0868, 2.2876) ccw projected
  line L67 (217.9385, 0.5719) -> (338.2351, 0.5719) projected
  arc A87 (338.2351, 0.5719) -> (357.9385, 0.5719) centre (348.0868, 2.2876) ccw projected
  line L68 (357.9385, 0.5719) -> (387.824, 0.5719) projected
  circle A88 centre (-146.9132, 65.5719) radius 11 projected
  line L69 (413.0868, 68.5719) -> (453.0868, 68.5719) projected
  arc A89 (453.0868, 62.5719) -> (453.0868, 68.5719) centre (453.0868, 65.5719) ccw projected
  line L70 (453.0868, 62.5719) -> (413.0868, 62.5719) projected
  arc A90 (413.0868, 68.5719) -> (413.0868, 62.5719) centre (413.0868, 65.5719) ccw projected
  circle A91 centre (-59.9132, 83.0715) radius 5.706
  circle A92 centre (58.0868, 90.5719) radius 2.5 projected
  circle A93 centre (58.0868, 90.5719) radius 7.5
  circle A94 centre (208.0868, 90.5719) radius 2.5 projected
  circle A95 centre (208.0868, 90.5719) radius 7.5
  circle A96 centre (82.4742, 8.0719) radius 2.5 projected
  circle A97 centre (82.4742, 8.0719) radius 5.812
  circle A98 centre (403.1957, 16.56) radius 2.5 projected
  circle A99 centre (403.1957, 16.56) radius 6.8911
  circle A100 centre (366.2493, 83.0719) radius 2.5 projected
  circle A101 centre (366.2493, 83.0719) radius 6.6319
  point P0 (0, 0)
  constraints: 6 centre point, 6 coincident
extrude "Extrusion3" add sketch "Sketch9" against normal up to surface (5 mm away) contours A61 | A62 | A66 | A68 | A71 | A73 | A95 A81 | A93 A82 | A91 | A97 | A99 | A101